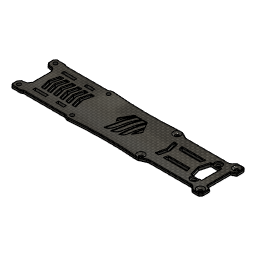
top_plate (Autodesk Fusion 360 design; units mm, degrees)
Autodesk Fusion 360 part; units mm, degrees
sketch "Sketch1" plane through (0, 0, 0) normal (0, 1, 0) x (1, 0, 0)
  line L0 (-47.713519, 13.1) -> (-47.713519, 11) construction
  line L1 (-41.213519, 13.1) -> (-41.213519, 11)
  line L2 (-56.590739, 11) -> (-67.090739, 11)
  line L3 (-67.090739, 11) -> (-67.090739, 13.1) construction
  line L4 (-47.713519, 11) -> (-47.713519, 13.1)
  line L5 (-41.213519, 11) -> (-47.713519, 11)
  line L6 (-56.590739, 11) -> (-67.090739, 11) construction
  line L7 (-67.090739, 13.1) -> (-56.590739, 13.1)
  line L8 (-47.713519, 13.1) -> (-41.213519, 13.1)
  line L9 (-56.590739, 13.1) -> (-56.590739, 11) construction
  line L10 (-41.213519, 11) -> (-41.213519, 13.1) construction
  line L11 (-41.213519, 13.1) -> (-47.713519, 13.1) construction
  line L12 (-47.713519, 11) -> (-41.213519, 11) construction
  line L13 (-56.590739, 13.1) -> (-56.590739, 11)
  line L14 (-67.090739, 11) -> (-67.090739, 13.1)
  line L15 (-67.090739, 13.1) -> (-56.590739, 13.1) construction
  line L16 (-70.174123, -18.17214) -> (-35.363156, -18.17214)
  arc A0 (25.451249, -18.878806) -> (-31.294288, -19.317303) centre (-0.303053, -357.951466) ccw
  line L17 (-78.946682, -19.052221) -> (-80.512717, -17.204486)
  line L18 (-80.512717, -17.204486) -> (-80.512717, -13.453934)
  line L19 (-80.512717, -13.453934) -> (-78.678868, -11.179487)
  line L20 (-72.154306, -19.052221) -> (-70.174123, -18.17214)
  line L21 (-78.678868, -11.179487) -> (-74.630702, -10.449798)
  line L22 (-41.21352, -11.000003) -> (-41.21352, -13.100003) construction
  line L23 (-47.71352, -11.000002) -> (-41.21352, -11.000003) construction
  line L24 (-41.21352, -13.100003) -> (-41.21352, -11.000003)
  line L25 (-47.71352, -13.100002) -> (-47.71352, -11.000002) construction
  line L26 (-56.59074, -11.000002) -> (-67.09074, -11.000001) construction
  line L27 (-41.21352, -13.100003) -> (-47.71352, -13.100002) construction
  line L28 (-56.59074, -13.100002) -> (-56.59074, -11.000002)
  line L29 (-67.09074, -13.100001) -> (-56.59074, -13.100002) construction
  line L30 (-67.09074, -13.100001) -> (-56.59074, -13.100002)
  line L31 (-47.71352, -11.000002) -> (-47.71352, -13.100002)
  line L32 (-41.21352, -11.000003) -> (-47.71352, -11.000002)
  line L33 (-56.59074, -11.000002) -> (-67.09074, -11.000001)
  line L34 (-56.59074, -13.100002) -> (-56.59074, -11.000002) construction
  line L35 (-47.71352, -13.100002) -> (-41.21352, -13.100003)
  line L36 (-67.09074, -11.000001) -> (-67.09074, -13.100001) construction
  line L37 (-67.09074, -11.000001) -> (-67.09074, -13.100001)
  circle A1 centre (-76.676945, -15.351861) radius 1.525
  line L38 (-74.630702, -10.449798) -> (-72.890045, -7.871569)
  line L39 (-78.946682, -19.052221) -> (-72.154306, -19.052221)
  line L40 (-72.890045, -7.871569) -> (-72.890045, 0.169525)
  circle A2 centre (-31.717186, 15.362679) radius 1.525
  circle A3 centre (-31.717186, -15.362679) radius 1.525
  circle A4 centre (26.228655, -15.29613) radius 1.525
  circle A5 centre (26.228655, 15.29613) radius 1.525
  arc A6 (-33.943222, -18.617483) -> (-35.363156, -18.17214) centre (-35.363156, -20.658473) ccw
  arc A7 (-33.943222, -18.617483) -> (-31.294288, -19.317303) centre (-31.658838, -15.33395) ccw
  line L41 (77.06033, 9.723206) -> (77.06033, 0)
  line L42 (80.674374, 17.200256) -> (80.667697, 11.53485)
  circle A8 centre (76.676945, 15.351861) radius 1.525
  line L43 (80.667697, 11.53485) -> (77.06033, 9.723206)
  line L44 (79.028958, 19.274953) -> (80.674374, 17.200256)
  line L45 (74.313283, 19.274953) -> (79.028958, 19.274953)
  line L46 (72.103018, 17.913723) -> (72.917518, 18.707378)
  line L47 (0, 0) -> (17, 0) construction
  arc A9 (-31.294288, 19.317303) -> (25.89772, 18.913013) centre (-0.303053, 357.951466) ccw
  arc A10 (-35.363156, 18.17214) -> (-33.943222, 18.617483) centre (-35.363156, 20.658473) ccw
  arc A11 (-31.294288, 19.317303) -> (-33.943222, 18.617483) centre (-31.658838, 15.33395) ccw
  line L48 (-70.174123, 18.17214) -> (-35.363156, 18.17214)
  line L49 (-72.154306, 19.052221) -> (-70.174123, 18.17214)
  line L50 (-72.890045, 7.871569) -> (-72.890045, -0.169525)
  line L51 (-78.678868, 11.179487) -> (-74.630702, 10.449798)
  line L52 (-80.512717, 13.453934) -> (-78.678868, 11.179487)
  line L53 (-74.630702, 10.449798) -> (-72.890045, 7.871569)
  circle A12 centre (-76.676945, 15.351861) radius 1.525
  line L54 (-78.946682, 19.052221) -> (-72.154306, 19.052221)
  line L55 (-80.512717, 17.204486) -> (-80.512717, 13.453934)
  line L56 (-78.946682, 19.052221) -> (-80.512717, 17.204486)
  line L57 (74.313283, -19.274953) -> (79.028958, -19.274953)
  line L58 (80.667697, -11.53485) -> (77.06033, -9.723206)
  line L59 (79.028958, -19.274953) -> (80.674374, -17.200256)
  line L60 (80.674374, -17.200256) -> (80.667697, -11.53485)
  line L61 (72.103018, -17.913723) -> (72.917518, -18.707378)
  circle A13 centre (76.676945, -15.351861) radius 1.525
  line L62 (77.06033, -9.723206) -> (77.06033, 0)
  line L63 (27.994774, 18.502613) -> (32.155418, 16.422291)
  line L64 (33.944272, 16) -> (68.977563, 16)
  line L65 (72.009935, 17.752225) -> (72.103018, 17.913723)
  line L66 (33.863514, -16) -> (68.977563, -16)
  line L67 (72.009935, -17.752225) -> (72.103018, -17.913723)
  line L68 (27.404322, -18.534068) -> (32.213389, -16.356227)
  arc A14 (27.994774, 18.502613) -> (25.89772, 18.913013) centre (26.20592, 14.924905) ccw
  arc A15 (32.155418, 16.422291) -> (33.944272, 16) centre (33.944272, 20) ccw
  arc A16 (33.863514, -16) -> (32.213389, -16.356227) centre (33.863514, -20) ccw
  arc A17 (25.451249, -18.878806) -> (27.404322, -18.534068) centre (25.754197, -14.890295) ccw
  arc A18 (68.977563, 16) -> (72.009935, 17.752225) centre (68.977563, 19.5) ccw
  arc A19 (72.009935, -17.752225) -> (68.977563, -16) centre (68.977563, -19.5) ccw
  arc A20 (74.313283, 19.274953) -> (72.917518, 18.707378) centre (74.313283, 17.274953) ccw
  arc A21 (72.917518, -18.707378) -> (74.313283, -19.274953) centre (74.313283, -17.274953) ccw
  point P0 (-76.676945, -15.351861)
  point P1 (-86.248614, -12.852519)
  point P2 (-76.676945, 15.351861)
  dimension "d36" = 10.5
  dimension "d37" = 2.1
  dimension "d38" = 6.5
  dimension "d39" = 2.1
  dimension "d132" = 4
  dimension "d144" = 4
  dimension "d145" = 4
  dimension "d146" = 4
  dimension "d147" = 4
  dimension "d148" = 3.5
  dimension "d149" = 3.5
  dimension "d150" = 2
  dimension "d151" = 2
  constraint horizontal L15
  constraint vertical L9
  constraint horizontal L6
  constraint vertical L3
  constraint horizontal L12
  constraint vertical L10
  constraint horizontal L11
  constraint vertical L0
  constraint horizontal L7
  constraint vertical L13
  constraint horizontal L2
  constraint vertical L14
  constraint horizontal L8
  constraint vertical L1
  constraint horizontal L5
  constraint vertical L4
  constraint vertical L40
  constraint horizontal L16
  constraint tangent L16 A6
  constraint tangent A0 A7
  constraint tangent A6 A7
  constraint coincident L47.start origin
  constraint horizontal L47
  constraint symmetric A0 L47 A9
  constraint symmetric A1 L47 A12
  constraint symmetric A6 L47 A10
  constraint symmetric A7 L47 A11
  constraint symmetric A8 L47 A13
  constraint vertical L62
  constraint tangent A9 A14
  constraint tangent L63 A14
  constraint tangent L63 A15
  constraint tangent L64 A15
  constraint tangent L68 A16
  constraint tangent L66 A16
  constraint tangent A0 A17
  constraint tangent L68 A17
  constraint tangent L65 A18
  constraint tangent L64 A18
  constraint tangent L67 A19
  constraint tangent L66 A19
  constraint tangent L46 A20
  constraint tangent L45 A20
  constraint tangent L61 A21
  constraint tangent L57 A21
  measures "d132" radius of A7
  measures "d144" radius of A14
  measures "d145" radius of A15
  measures "d146" radius of A16
  measures "d147" radius of A17
  measures "d148" radius of A18
  measures "d149" radius of A19
  measures "d150" radius of A20
  measures "d151" radius of A21
extrude "Extrude1" add sketch "Sketch1" along normal blind 2.5 contours L16 A0 L17 L18 L19 L20 L21 L38 L39 L40 A6 A7 L41 L42 L43 L44 L45 L46 A9 A10 A11 L48 L49 L50 L51 L52 L53 L54 L55 L56 L57 L58 L59 L60 L61 L62 L63 L64 L65 L66 L67 L68 A14 A15 A16 A17 A18 A19 A20 A21 picked at (45.595116, -5.333333)
sketch "Sketch2" plane through (0, 2.5, 0) normal (0, 1, 0) x (-1, 0, 0)
  line L0 (49.365614, -7.482923) -> (47.32507, -7.482923)
  line L1 (49.365614, 7.482923) -> (47.32507, 7.482923)
  line L2 (64.765331, -7.482923) -> (62.724788, -7.482923)
  line L3 (62.724788, 7.482923) -> (64.493676, 0)
  line L4 (57.769481, 7.482923) -> (59.538369, 0)
  line L5 (47.32507, 7.482923) -> (49.093958, 0)
  line L6 (47.32507, -7.482923) -> (49.093958, 0)
  line L7 (57.769481, -7.482923) -> (59.538369, 0)
  line L8 (57.769481, -7.482923) -> (59.538369, 0)
  line L9 (51.134502, 0) -> (49.365614, 7.482923)
  line L10 (47.32507, -7.482923) -> (49.093958, 0)
  line L11 (51.134502, 0) -> (49.365614, 7.482923)
  line L12 (62.724788, -7.482923) -> (64.493676, 0)
  line L13 (61.578913, 0) -> (59.810025, -7.482923)
  line L14 (49.365614, 7.482923) -> (47.32507, 7.482923)
  line L15 (66.534219, 0) -> (64.765331, -7.482923)
  line L16 (52.598933, -7.482923) -> (54.367821, 0)
  line L17 (51.134502, 0) -> (49.365614, -7.482923)
  line L18 (56.408365, 0) -> (54.639477, -7.482923)
  line L19 (51.134502, 0) -> (49.365614, -7.482923)
  line L20 (52.598933, -7.482923) -> (54.367821, 0)
  line L21 (47.32507, 7.482923) -> (49.093958, 0)
  line L22 (56.408365, 0) -> (54.639477, -7.482923)
  line L23 (61.578913, 0) -> (59.810025, -7.482923)
  line L24 (42.260502, 0) -> (17, 0) construction
  line L25 (59.810025, 7.482923) -> (57.769481, 7.482923)
  line L26 (59.810025, -7.482923) -> (57.769481, -7.482923)
  line L27 (64.765331, 7.482923) -> (62.724788, 7.482923)
  line L28 (61.578913, 0) -> (59.810025, 7.482923)
  line L29 (59.810025, 7.482923) -> (57.769481, 7.482923)
  line L30 (57.769481, 7.482923) -> (59.538369, 0)
  line L31 (59.810025, -7.482923) -> (57.769481, -7.482923)
  line L32 (49.365614, -7.482923) -> (47.32507, -7.482923)
  line L33 (56.408365, 0) -> (54.639477, 7.482923)
  line L34 (54.639477, 7.482923) -> (52.598933, 7.482923)
  line L35 (56.408365, 0) -> (54.639477, 7.482923)
  line L36 (66.534219, 0) -> (64.765331, 7.482923)
  line L37 (52.598933, 7.482923) -> (54.367821, 0)
  line L38 (54.639477, -7.482923) -> (52.598933, -7.482923)
  line L39 (61.578913, 0) -> (59.810025, 7.482923)
  line L40 (52.598933, 7.482923) -> (54.367821, 0)
  line L41 (54.639477, 7.482923) -> (52.598933, 7.482923)
  line L42 (54.639477, -7.482923) -> (52.598933, -7.482923)
  arc A0 (-25.451249, 18.878806) -> (31.294288, 19.317303) centre (0.303053, 357.951466) ccw
  line L43 (74.630702, 10.449798) -> (78.678868, 11.179487)
  line L44 (78.678868, 11.179487) -> (80.512717, 13.453934)
  line L45 (80.512717, 13.453934) -> (80.512717, 17.204486)
  line L46 (80.512717, 17.204486) -> (78.946682, 19.052221)
  line L47 (67.09074, 13.100001) -> (67.09074, 11.000001)
  line L48 (67.09074, 11.000001) -> (56.59074, 11.000002)
  line L49 (56.59074, 11.000002) -> (56.59074, 13.100002)
  line L50 (56.59074, 13.100002) -> (67.09074, 13.100001)
  line L51 (41.21352, 13.100003) -> (47.71352, 13.100002)
  line L52 (47.71352, 13.100002) -> (47.71352, 11.000002)
  line L53 (47.71352, 11.000002) -> (41.21352, 11.000003)
  line L54 (41.21352, 11.000003) -> (41.21352, 13.100003)
  line L55 (0, 0) -> (0, -25) construction
  line L56 (45.963858, 0) -> (44.19497, -7.482923)
  line L57 (42.154426, 7.482923) -> (43.923314, 0)
  line L58 (44.19497, -7.482923) -> (42.154426, -7.482923)
  line L59 (42.154426, 7.482923) -> (43.923314, 0)
  line L60 (38.921107, -7.482923) -> (36.880563, -7.482923)
  line L61 (44.19497, 7.482923) -> (42.154426, 7.482923)
  line L62 (36.880563, 7.482923) -> (38.649451, 0)
  line L63 (40.689995, 0) -> (38.921107, -7.482923)
  line L64 (40.689995, 0) -> (38.921107, 7.482923)
  line L65 (36.880563, -7.482923) -> (38.649451, 0)
  line L66 (45.963858, 0) -> (44.19497, 7.482923)
  line L67 (45.963858, 0) -> (44.19497, -7.482923)
  line L68 (38.921107, 7.482923) -> (36.880563, 7.482923)
  line L69 (42.154426, -7.482923) -> (43.923314, 0)
  line L70 (40.689995, 0) -> (38.921107, -7.482923)
  line L71 (40.689995, 0) -> (38.921107, 7.482923)
  line L72 (45.963858, 0) -> (44.19497, 7.482923)
  line L73 (38.921107, 7.482923) -> (36.880563, 7.482923)
  line L74 (36.880563, -7.482923) -> (38.649451, 0)
  line L75 (38.921107, -7.482923) -> (36.880563, -7.482923)
  line L76 (44.19497, -7.482923) -> (42.154426, -7.482923)
  line L77 (44.19497, 7.482923) -> (42.154426, 7.482923)
  line L78 (42.154426, -7.482923) -> (43.923314, 0)
  line L79 (36.880563, 7.482923) -> (38.649451, 0)
  line L80 (56.590739, -11) -> (67.090739, -11)
  line L81 (67.090739, -11) -> (67.090739, -13.1)
  line L82 (67.090739, -13.1) -> (56.590739, -13.1)
  line L83 (56.590739, -13.1) -> (56.590739, -11)
  line L84 (47.713519, -11) -> (47.713519, -13.1)
  line L85 (47.713519, -13.1) -> (41.213519, -13.1)
  line L86 (41.213519, -13.1) -> (41.213519, -11)
  line L87 (41.213519, -11) -> (47.713519, -11)
  line L88 (3.784933, -10.888484) -> (5.164029, -10.888484)
  line L89 (5.164029, -10.888484) -> (10.465412, -1.792331)
  line L90 (10.465412, -1.792331) -> (8.908366, 0.941707)
  spline S0 degree 2 poles (8.908366, 0.941707) (7.442966, -3.619944) (6.490839, -5.818435) knots 0 0 0 1 1 1
  spline S1 degree 2 poles (6.490839, -5.818435) (5.538712, -8.01694) (3.784933, -10.888484) knots 0 0 0 1 1 1
  line L91 (3.0098, -10.88842) -> (-0.824674, -10.88842)
  spline S2 degree 2 poles (-0.824674, -10.88842) (1.360907, -6.965735) (2.348646, -3.92432) knots 0 0 0 1 1 1
  spline S3 degree 3 poles (2.348646, -3.92432) (2.771725, -2.621651) (3.140209, -0.972131) (3.497406, 0.716522) knots 0 0 0 0 1 1 1 1
  spline S4 degree 2 poles (3.497406, 0.716522) (4.23037, 4.1815) (4.970387, 6.954955) knots 0 0 0 1 1 1
  spline S5 degree 2 poles (4.970387, 6.954955) (5.912838, 8.886413) (6.686031, 9.591534) knots 0 0 0 1 1 1
  spline S6 degree 2 poles (6.686031, 9.591534) (7.45921, 10.296651) (9.286239, 10.890851) knots 0 0 0 1 1 1
  spline S7 degree 2 poles (9.286239, 10.890851) (8.697628, 8.517032) (8.444231, 7.377107) knots 0 0 0 1 1 1
  spline S8 degree 3 poles (8.444231, 7.377107) (7.319167, 2.315979) (6.475945, -1.46655) (5.82273, -3.733217) knots 0 0 0 0 1 1 1 1
  spline S9 degree 2 poles (5.82273, -3.733217) (4.622239, -7.89888) (3.0098, -10.88842) knots 0 0 0 1 1 1
  line L92 (-5.475454, -10.888568) -> (-1.57567, -10.888568)
  spline S10 degree 2 poles (-1.57567, -10.888568) (-0.309354, -8.857824) (0.803309, -4.528704) knots 0 0 0 1 1 1
  spline S11 degree 3 poles (0.803309, -4.528704) (1.40458, -2.189429) (2.133696, 1.762827) (3.137408, 6.936551) knots 0 0 0 0 1 1 1 1
  spline S12 degree 2 poles (3.137408, 6.936551) (3.371965, 8.145592) (3.947428, 10.600128) knots 0 0 0 1 1 1
  spline S13 degree 2 poles (3.947428, 10.600128) (1.954848, 9.817553) (1.208318, 9.274906) knots 0 0 0 1 1 1
  spline S14 degree 2 poles (1.208318, 9.274906) (0.461787, 8.732257) (-0.413542, 6.936551) knots 0 0 0 1 1 1
  spline S15 degree 3 poles (-0.413542, 6.936551) (-1.94327, -0.721308) (-2.284933, -2.657156) (-2.760299, -4.305109) knots 0 0 0 0 1 1 1 1
  spline S16 degree 2 poles (-2.760299, -4.305109) (-3.726791, -7.655622) (-5.475454, -10.888568) knots 0 0 0 1 1 1
  line L93 (-5.931273, -10.089814) -> (-8.252962, -6.117535)
  spline S17 degree 2 poles (-8.252962, -6.117535) (-7.281055, -3.828239) (-6.709183, -1.384106) knots 0 0 0 1 1 1
  spline S18 degree 3 poles (-6.709183, -1.384106) (-6.653776, -1.1473) (-6.602886, -0.909225) (-6.555659, -0.670152) knots 0 0 0 0 1 1 1 1
  spline S19 degree 2 poles (-6.555659, -0.670152) (-5.82338, 3.035977) (-5.475431, 6.081951) knots 0 0 0 1 1 1
  spline S20 degree 2 poles (-5.475431, 6.081951) (-4.761037, 7.878925) (-4.217823, 8.34514) knots 0 0 0 1 1 1
  spline S21 degree 2 poles (-4.217823, 8.34514) (-3.67461, 8.811357) (-1.998782, 9.685931) knots 0 0 0 1 1 1
  spline S22 degree 2 poles (-1.998782, 9.685931) (-2.82745, 1.291461) (-3.650811, -2.849077) knots 0 0 0 1 1 1
  spline S23 degree 2 poles (-3.650811, -2.849077) (-4.474167, -6.989544) (-5.931273, -10.089814) knots 0 0 0 1 1 1
  line L94 (-10.780246, -1.792357) -> (-8.746198, -5.184925)
  spline S24 degree 2 poles (-8.746198, -5.184925) (-8.089469, -2.881961) (-7.835471, -1.200861) knots 0 0 0 1 1 1
  spline S25 degree 2 poles (-7.835471, -1.200861) (-7.581474, 0.480239) (-7.336445, 4.14564) knots 0 0 0 1 1 1
  spline S26 degree 2 poles (-7.336445, 4.14564) (-8.484273, 2.354181) (-9.058345, 1.364332) knots 0 0 0 1 1 1
  spline S27 degree 2 poles (-9.058345, 1.364332) (-9.632426, 0.374469) (-10.780246, -1.792357) knots 0 0 0 1 1 1
  line L95 (56.540739, -10.95) -> (67.140739, -10.95)
  line L96 (67.140739, -10.95) -> (67.140739, -13.15)
  line L97 (67.140739, -13.15) -> (56.540739, -13.15)
  line L98 (56.540739, -13.15) -> (56.540739, -10.95)
  line L99 (41.163519, -10.95) -> (47.763519, -10.95)
  line L100 (47.763519, -10.95) -> (47.763519, -13.15)
  line L101 (47.763519, -13.15) -> (41.163519, -13.15)
  line L102 (41.163519, -13.15) -> (41.163519, -10.95)
  line L103 (56.54074, 13.150002) -> (67.14074, 13.150001)
  line L104 (67.14074, 13.150001) -> (67.14074, 10.950001)
  line L105 (67.14074, 10.950001) -> (56.54074, 10.950002)
  line L106 (56.54074, 10.950002) -> (56.54074, 13.150002)
  line L107 (41.16352, 13.150003) -> (47.76352, 13.150002)
  line L108 (47.76352, 13.150002) -> (47.76352, 10.950002)
  line L109 (47.76352, 10.950002) -> (41.16352, 10.950003)
  line L110 (41.16352, 10.950003) -> (41.16352, 13.150003)
  line L111 (72.154306, -19.052221) -> (78.946682, -19.052221)
  line L112 (78.946682, -19.052221) -> (80.512717, -17.204486)
  line L113 (80.512717, -17.204486) -> (80.512717, -13.453934)
  line L114 (80.512717, -13.453934) -> (78.678868, -11.179487)
  line L115 (78.678868, -11.179487) -> (74.630702, -10.449798)
  line L116 (74.630702, -10.449798) -> (72.890045, -7.871569)
  line L117 (72.890045, -7.871569) -> (72.890045, 7.871569)
  line L118 (72.890045, 7.871569) -> (74.630702, 10.449798)
  line L119 (78.946682, 19.052221) -> (72.154306, 19.052221)
  line L120 (72.154306, 19.052221) -> (70.174123, 18.17214)
  line L121 (70.174123, 18.17214) -> (35.363156, 18.17214)
  arc A1 (33.943222, 18.617483) -> (35.363156, 18.17214) centre (35.363156, 20.658473) ccw
  arc A2 (33.943222, 18.617483) -> (31.294288, 19.317303) centre (31.658838, 15.33395) ccw
  line L122 (-77.06033, -9.723206) -> (-80.667697, -11.53485)
  line L123 (-80.667697, -11.53485) -> (-80.674374, -17.200256)
  line L124 (-80.674374, -17.200256) -> (-79.028958, -19.274953)
  line L125 (-79.028958, -19.274953) -> (-74.313283, -19.274953)
  line L126 (-72.917518, -18.707378) -> (-72.103018, -17.913723)
  arc A3 (31.294288, -19.317303) -> (-25.89772, -18.913013) centre (0.303053, -357.951466) ccw
  arc A4 (31.294288, -19.317303) -> (33.943222, -18.617483) centre (31.658838, -15.33395) ccw
  arc A5 (35.363156, -18.17214) -> (33.943222, -18.617483) centre (35.363156, -20.658473) ccw
  line L127 (35.363156, -18.17214) -> (70.174123, -18.17214)
  line L128 (70.174123, -18.17214) -> (72.154306, -19.052221)
  line L129 (-72.103018, 17.913723) -> (-72.917518, 18.707378)
  line L130 (-74.313283, 19.274953) -> (-79.028958, 19.274953)
  line L131 (-79.028958, 19.274953) -> (-80.674374, 17.200256)
  line L132 (-80.674374, 17.200256) -> (-80.667697, 11.53485)
  line L133 (-80.667697, 11.53485) -> (-77.06033, 9.723206)
  line L134 (-77.06033, 9.723206) -> (-77.06033, -9.723206)
  circle A6 centre (76.676945, 15.351861) radius 1.525
  circle A7 centre (-76.676945, -15.351861) radius 1.525
  circle A8 centre (-26.228655, -15.29613) radius 1.525
  circle A9 centre (31.717186, -15.362679) radius 1.525
  circle A10 centre (31.717186, 15.362679) radius 1.525
  circle A11 centre (-26.228655, 15.29613) radius 1.525
  circle A12 centre (76.676945, -15.351861) radius 1.525
  circle A13 centre (-76.676945, 15.351861) radius 1.525
  line L135 (-57.244978, 7.438362) -> (-38.408116, 7.438362)
  line L136 (-39.09255, 4.935443) -> (-56.560544, 4.935443)
  line L137 (-38.408116, -7.438362) -> (-57.244978, -7.438362)
  line L138 (-56.560544, -4.935443) -> (-39.09255, -4.935443)
  line L139 (-56.560544, 4.935443) -> (-57.244978, 7.438362)
  line L140 (-57.244978, -7.438362) -> (-56.560544, -4.935443)
  line L141 (-38.408116, 7.438362) -> (-39.09255, 4.935443)
  line L142 (-39.09255, -4.935443) -> (-38.408116, -7.438362)
  line L143 (-35.348965, 0) -> (-33.580077, 7.482923)
  line L144 (-31.539534, 7.482923) -> (-33.308422, 0)
  line L145 (-33.580077, 7.482923) -> (-31.539534, 7.482923)
  line L146 (-33.580077, -7.482923) -> (-35.348965, 0)
  line L147 (-33.308422, 0) -> (-31.539534, -7.482923)
  line L148 (-31.539534, -7.482923) -> (-33.580077, -7.482923)
  line L149 (-27.404322, 18.534068) -> (-32.213389, 16.356227)
  line L150 (-33.863514, 16) -> (-68.977563, 16)
  line L151 (-72.009935, 17.752225) -> (-72.103018, 17.913723)
  line L152 (-72.103018, -17.913723) -> (-72.009935, -17.752225)
  line L153 (-68.977563, -16) -> (-33.944272, -16)
  line L154 (-32.155418, -16.422291) -> (-27.994774, -18.502613)
  arc A14 (-25.451249, 18.878806) -> (-27.404322, 18.534068) centre (-25.754197, 14.890295) ccw
  arc A15 (-33.863514, 16) -> (-32.213389, 16.356227) centre (-33.863514, 20) ccw
  arc A16 (-32.155418, -16.422291) -> (-33.944272, -16) centre (-33.944272, -20) ccw
  arc A17 (-27.994774, -18.502613) -> (-25.89772, -18.913013) centre (-26.20592, -14.924905) ccw
  arc A18 (-72.917518, 18.707378) -> (-74.313283, 19.274953) centre (-74.313283, 17.274953) ccw
  arc A19 (-74.313283, -19.274953) -> (-72.917518, -18.707378) centre (-74.313283, -17.274953) ccw
  arc A20 (-68.977563, -16) -> (-72.009935, -17.752225) centre (-68.977563, -19.5) ccw
  arc A21 (-72.009935, 17.752225) -> (-68.977563, 16) centre (-68.977563, 19.5) ccw
  point P0 (66.429305, 0)
  point P1 (66.429305, 0)
  dimension "d110" = -0.05
  dimension "d111" = -0.05
  dimension "d112" = -0.05
  dimension "d113" = -0.05
  constraint horizontal L2
  constraint parallel L12 L15
  constraint horizontal L26
  constraint parallel L7 L13
  constraint horizontal L31
  constraint parallel L8 L23
  constraint horizontal L38
  constraint parallel L16 L22
  constraint horizontal L42
  constraint parallel L18 L20
  constraint horizontal L32
  constraint parallel L6 L19
  constraint horizontal L0
  constraint parallel L10 L17
  constraint coincident L55.start origin
  constraint horizontal L76
  constraint parallel L56 L69
  constraint horizontal L58
  constraint parallel L67 L78
  constraint horizontal L75
  constraint parallel L63 L74
  constraint horizontal L60
  constraint parallel L65 L70
sketch "Sketch3" plane through (0, 2.5, 0) normal (0, 1, 0) x (-1, 0, 0)
  arc A0 (-25.451249, 18.878806) -> (31.294288, 19.317303) centre (0.303053, 357.951466) ccw
  line L0 (74.630702, 10.449798) -> (78.678868, 11.179487)
  line L1 (78.678868, 11.179487) -> (80.512717, 13.453934)
  line L2 (80.512717, 13.453934) -> (80.512717, 17.204486)
  line L3 (80.512717, 17.204486) -> (78.946682, 19.052221)
  line L4 (67.09074, 13.100001) -> (67.09074, 11.000001)
  line L5 (67.09074, 11.000001) -> (56.59074, 11.000002)
  line L6 (56.59074, 11.000002) -> (56.59074, 13.100002)
  line L7 (56.59074, 13.100002) -> (67.09074, 13.100001)
  line L8 (41.21352, 13.100003) -> (47.71352, 13.100002)
  line L9 (47.71352, 13.100002) -> (47.71352, 11.000002)
  line L10 (47.71352, 11.000002) -> (41.21352, 11.000003)
  line L11 (41.21352, 11.000003) -> (41.21352, 13.100003)
  line L12 (56.590739, -11) -> (67.090739, -11)
  line L13 (67.090739, -11) -> (67.090739, -13.1)
  line L14 (67.090739, -13.1) -> (56.590739, -13.1)
  line L15 (56.590739, -13.1) -> (56.590739, -11)
  line L16 (47.713519, -11) -> (47.713519, -13.1)
  line L17 (47.713519, -13.1) -> (41.213519, -13.1)
  line L18 (41.213519, -13.1) -> (41.213519, -11)
  line L19 (41.213519, -11) -> (47.713519, -11)
  line L20 (72.154306, -19.052221) -> (78.946682, -19.052221)
  line L21 (78.946682, -19.052221) -> (80.512717, -17.204486)
  line L22 (80.512717, -17.204486) -> (80.512717, -13.453934)
  line L23 (80.512717, -13.453934) -> (78.678868, -11.179487)
  line L24 (78.678868, -11.179487) -> (74.630702, -10.449798)
  line L25 (74.630702, -10.449798) -> (72.890045, -7.871569)
  line L26 (72.890045, -7.871569) -> (72.890045, 7.871569)
  line L27 (72.890045, 7.871569) -> (74.630702, 10.449798)
  line L28 (78.946682, 19.052221) -> (72.154306, 19.052221)
  line L29 (72.154306, 19.052221) -> (70.174123, 18.17214)
  line L30 (70.174123, 18.17214) -> (35.363156, 18.17214)
  arc A1 (33.943222, 18.617483) -> (35.363156, 18.17214) centre (35.363156, 20.658473) ccw
  arc A2 (33.943222, 18.617483) -> (31.294288, 19.317303) centre (31.658838, 15.33395) ccw
  line L31 (-77.06033, -9.723206) -> (-80.667697, -11.53485)
  line L32 (-80.667697, -11.53485) -> (-80.674374, -17.200256)
  line L33 (-80.674374, -17.200256) -> (-79.028958, -19.274953)
  line L34 (-79.028958, -19.274953) -> (-74.313283, -19.274953)
  line L35 (-72.917518, -18.707378) -> (-72.103018, -17.913723)
  arc A3 (31.294288, -19.317303) -> (-25.89772, -18.913013) centre (0.303053, -357.951466) ccw
  arc A4 (31.294288, -19.317303) -> (33.943222, -18.617483) centre (31.658838, -15.33395) ccw
  arc A5 (35.363156, -18.17214) -> (33.943222, -18.617483) centre (35.363156, -20.658473) ccw
  line L36 (35.363156, -18.17214) -> (70.174123, -18.17214)
  line L37 (70.174123, -18.17214) -> (72.154306, -19.052221)
  line L38 (-72.103018, 17.913723) -> (-72.917518, 18.707378)
  line L39 (-74.313283, 19.274953) -> (-79.028958, 19.274953)
  line L40 (-79.028958, 19.274953) -> (-80.674374, 17.200256)
  line L41 (-80.674374, 17.200256) -> (-80.667697, 11.53485)
  line L42 (-80.667697, 11.53485) -> (-77.06033, 9.723206)
  line L43 (-77.06033, 9.723206) -> (-77.06033, -9.723206)
  circle A6 centre (76.676945, 15.351861) radius 1.525
  circle A7 centre (-76.676945, -15.351861) radius 1.525
  circle A8 centre (-26.228655, -15.29613) radius 1.525
  circle A9 centre (31.717186, -15.362679) radius 1.525
  circle A10 centre (31.717186, 15.362679) radius 1.525
  circle A11 centre (-26.228655, 15.29613) radius 1.525
  circle A12 centre (76.676945, -15.351861) radius 1.525
  circle A13 centre (-76.676945, 15.351861) radius 1.525
  line L44 (-27.404322, 18.534068) -> (-32.213389, 16.356227)
  line L45 (-33.863514, 16) -> (-68.977563, 16)
  line L46 (-72.009935, 17.752225) -> (-72.103018, 17.913723)
  line L47 (-72.103018, -17.913723) -> (-72.009935, -17.752225)
  line L48 (-68.977563, -16) -> (-33.944272, -16)
  line L49 (-32.155418, -16.422291) -> (-27.994774, -18.502613)
  arc A14 (-25.451249, 18.878806) -> (-27.404322, 18.534068) centre (-25.754197, 14.890295) ccw
  arc A15 (-33.863514, 16) -> (-32.213389, 16.356227) centre (-33.863514, 20) ccw
  arc A16 (-32.155418, -16.422291) -> (-33.944272, -16) centre (-33.944272, -20) ccw
  arc A17 (-27.994774, -18.502613) -> (-25.89772, -18.913013) centre (-26.20592, -14.924905) ccw
  arc A18 (-72.917518, 18.707378) -> (-74.313283, 19.274953) centre (-74.313283, 17.274953) ccw
  arc A19 (-74.313283, -19.274953) -> (-72.917518, -18.707378) centre (-74.313283, -17.274953) ccw
  arc A20 (-68.977563, -16) -> (-72.009935, -17.752225) centre (-68.977563, -19.5) ccw
  arc A21 (-72.009935, 17.752225) -> (-68.977563, 16) centre (-68.977563, 19.5) ccw
sketch "Sketch4" plane through (0, 2.5, 0) normal (0, 1, 0) x (-1, 0, 0)
  line L0 (67.09074, 13.100001) -> (67.09074, 11.000001)
  line L1 (67.09074, 11.000001) -> (56.59074, 11.000002)
  line L2 (56.59074, 11.000002) -> (56.59074, 13.100002)
  line L3 (56.59074, 13.100002) -> (67.09074, 13.100001)
  line L4 (41.21352, 13.100003) -> (47.71352, 13.100002)
  line L5 (47.71352, 13.100002) -> (47.71352, 11.000002)
  line L6 (47.71352, 11.000002) -> (41.21352, 11.000003)
  line L7 (41.21352, 11.000003) -> (41.21352, 13.100003)
  line L8 (74.630702, 10.449798) -> (78.678868, 11.179487)
  line L9 (78.678868, 11.179487) -> (80.512717, 13.453934)
  line L10 (80.512717, 13.453934) -> (80.512717, 17.204486)
  line L11 (80.512717, 17.204486) -> (78.946682, 19.052221)
  arc A0 (-25.451249, 18.878806) -> (31.294288, 19.317303) centre (0.303053, 357.951466) ccw
  line L12 (56.590739, -11) -> (67.090739, -11)
  line L13 (67.090739, -11) -> (67.090739, -13.1)
  line L14 (67.090739, -13.1) -> (56.590739, -13.1)
  line L15 (56.590739, -13.1) -> (56.590739, -11)
  line L16 (47.713519, -11) -> (47.713519, -13.1)
  line L17 (47.713519, -13.1) -> (41.213519, -13.1)
  line L18 (41.213519, -13.1) -> (41.213519, -11)
  line L19 (41.213519, -11) -> (47.713519, -11)
  line L20 (72.154306, -19.052221) -> (78.946682, -19.052221)
  line L21 (78.946682, -19.052221) -> (80.512717, -17.204486)
  line L22 (80.512717, -17.204486) -> (80.512717, -13.453934)
  line L23 (80.512717, -13.453934) -> (78.678868, -11.179487)
  line L24 (78.678868, -11.179487) -> (74.630702, -10.449798)
  line L25 (74.630702, -10.449798) -> (72.890045, -7.871569)
  line L26 (72.890045, -7.871569) -> (72.890045, 7.871569)
  line L27 (72.890045, 7.871569) -> (74.630702, 10.449798)
  line L28 (78.946682, 19.052221) -> (72.154306, 19.052221)
  line L29 (72.154306, 19.052221) -> (70.174123, 18.17214)
  line L30 (70.174123, 18.17214) -> (35.363156, 18.17214)
  arc A1 (33.943222, 18.617483) -> (35.363156, 18.17214) centre (35.363156, 20.658473) ccw
  arc A2 (33.943222, 18.617483) -> (31.294288, 19.317303) centre (31.658838, 15.33395) ccw
  line L31 (-77.06033, -9.723206) -> (-80.667697, -11.53485)
  line L32 (-80.667697, -11.53485) -> (-80.674374, -17.200256)
  line L33 (-80.674374, -17.200256) -> (-79.028958, -19.274953)
  line L34 (-79.028958, -19.274953) -> (-74.313283, -19.274953)
  line L35 (-72.917518, -18.707378) -> (-72.103018, -17.913723)
  arc A3 (31.294288, -19.317303) -> (-25.89772, -18.913013) centre (0.303053, -357.951466) ccw
  arc A4 (31.294288, -19.317303) -> (33.943222, -18.617483) centre (31.658838, -15.33395) ccw
  arc A5 (35.363156, -18.17214) -> (33.943222, -18.617483) centre (35.363156, -20.658473) ccw
  line L36 (35.363156, -18.17214) -> (70.174123, -18.17214)
  line L37 (70.174123, -18.17214) -> (72.154306, -19.052221)
  line L38 (-72.103018, 17.913723) -> (-72.917518, 18.707378)
  line L39 (-74.313283, 19.274953) -> (-79.028958, 19.274953)
  line L40 (-79.028958, 19.274953) -> (-80.674374, 17.200256)
  line L41 (-80.674374, 17.200256) -> (-80.667697, 11.53485)
  line L42 (-80.667697, 11.53485) -> (-77.06033, 9.723206)
  line L43 (-77.06033, 9.723206) -> (-77.06033, -9.723206)
  circle A6 centre (76.676945, 15.351861) radius 1.525
  circle A7 centre (-76.676945, -15.351861) radius 1.525
  circle A8 centre (-26.228655, -15.29613) radius 1.525
  circle A9 centre (31.717186, -15.362679) radius 1.525
  circle A10 centre (31.717186, 15.362679) radius 1.525
  circle A11 centre (-26.228655, 15.29613) radius 1.525
  circle A12 centre (76.676945, -15.351861) radius 1.525
  circle A13 centre (-76.676945, 15.351861) radius 1.525
  line L44 (-70.347842, 8.00136) -> (-62.171638, 8.00136)
  line L45 (-62.171638, 8.00136) -> (-62.171638, -7.99864)
  line L46 (-62.171638, -7.99864) -> (-70.347842, -7.99864)
  line L47 (-70.347842, -7.99864) -> (-70.347842, 8.00136)
  line L48 (-70.347842, 8.00136) -> (-62.171638, -7.99864) construction
  line L49 (-62.171638, 8.00136) -> (-70.347842, -7.99864) construction
  line L50 (-66.25974, 0.00136) -> (-66.25974, 10.25136) construction
  circle A14 centre (-66.25974, 10.25136) radius 1.5
  line L51 (-66.25974, 0.00136) -> (-68.381403, 0.00136) construction
  arc A15 (-68.150847, 7.872763) -> (-67.537373, 9.089722) centre (-68.175066, 8.648079) ccw
  arc A16 (-65.14647, 9.109265) -> (-64.491693, 7.787577) centre (-64.452409, 8.630074) ccw
  line L52 (-27.404322, 18.534068) -> (-32.213389, 16.356227)
  line L53 (-33.863514, 16) -> (-68.977563, 16)
  line L54 (-72.009935, 17.752225) -> (-72.103018, 17.913723)
  line L55 (-72.103018, -17.913723) -> (-72.009935, -17.752225)
  line L56 (-68.977563, -16) -> (-33.944272, -16)
  line L57 (-32.155418, -16.422291) -> (-27.994774, -18.502613)
  arc A17 (-25.451249, 18.878806) -> (-27.404322, 18.534068) centre (-25.754197, 14.890295) ccw
  arc A18 (-33.863514, 16) -> (-32.213389, 16.356227) centre (-33.863514, 20) ccw
  arc A19 (-32.155418, -16.422291) -> (-33.944272, -16) centre (-33.944272, -20) ccw
  arc A20 (-27.994774, -18.502613) -> (-25.89772, -18.913013) centre (-26.20592, -14.924905) ccw
  arc A21 (-72.917518, 18.707378) -> (-74.313283, 19.274953) centre (-74.313283, 17.274953) ccw
  arc A22 (-74.313283, -19.274953) -> (-72.917518, -18.707378) centre (-74.313283, -17.274953) ccw
  arc A23 (-68.977563, -16) -> (-72.009935, -17.752225) centre (-68.977563, -19.5) ccw
  arc A24 (-72.009935, 17.752225) -> (-68.977563, 16) centre (-68.977563, 19.5) ccw
  line L58 (-62.171638, 8.00136) -> (-59.908914, 0.070882)
  line L59 (-59.908914, 0.070882) -> (-62.171638, -7.99864)
  circle A25 centre (-66.25974, 10.25136) radius 3.1
  circle A26 centre (-66.25974, -10.24864) radius 3.1
  arc A27 (-64.491693, -7.784856) -> (-65.14647, -9.106544) centre (-64.452409, -8.627354) ccw
  arc A28 (-67.537373, -9.087001) -> (-68.150847, -7.870042) centre (-68.175066, -8.645358) ccw
  circle A29 centre (-66.25974, -10.24864) radius 1.5
  point P0 (-66.25974, 0.00136)
  point P1 (-66.25974, -10.24864)
  dimension "d136" = 16
  dimension "d139" = 3
  dimension "d155" = 6.2
  dimension "d159" = 10.25
  dimension "d160" = 16
  constraint horizontal L44
  constraint perpendicular L44 L45
  constraint parallel L45 L47
  constraint perpendicular L44 L50
  constraint perpendicular L50 L51
  constraint concentric A14 A25
  constraint symmetric A14 L51 A29
  constraint symmetric L51 A15 A28
  constraint symmetric L51 A16 A27
  constraint symmetric L51 A25 A26
  measures "d139" diameter of A14
  measures "d155" diameter of A25
hole "Hole2" at (26.228655, 2.5, -15.29613) at (26.228655, 2.5, 15.29613) at (76.676945, 2.5, 15.351861) at (76.676945, 2.5, -15.351861) direction (0, -1, 0) diameter 3.2 depth 4.760684 tip angle 118 countersink diameter 6.2 countersink angle 90
extrude "Extrude4" cut sketch "Sketch2" against normal blind 4.341 contours L95 L96 L97 L98 | L99 L100 L101 L102 | L103 L104 L105 L106 | L107 L108 L109 L110 | L135 L136 L139 L141 | L137 L138 L140 L142 | L143 L144 L145 L146 L147 L148 picked at (60.090739, -13.133333) picked at (43.380186, -13.133333) picked at (63.59074, 10.966668) picked at (45.546853, 10.966669) picked at (-44.915215, 6.604056) picked at (-44.915215, -6.604056) picked at (-32.809344, -4.988615)
extrude "Extrude6" cut sketch "Sketch2" against normal blind 10.279 contours L0 L1 L5 L6 L9 L10 L11 L14 L17 L19 L21 L32 | L2 L3 L12 L15 L27 L36 | L4 L7 L8 L13 L23 L25 L26 L28 L29 L30 L31 L39 | L16 L18 L20 L22 L33 L34 L35 L37 L38 L40 L41 L42 | L56 L57 L58 L59 L61 L66 L67 L69 L72 L76 L77 L78 | L60 L62 L63 L64 L65 L68 L70 L71 L73 L74 L75 L79 picked at (48.594881, -4.988615) picked at (63.994598, -4.988615) picked at (59.039292, -4.988615) picked at (53.868744, -4.988615) picked at (44.694047, -2.494308) picked at (38.150374, -4.988615)
extrude "Extrude8" cut sketch "Sketch4" against normal blind 3.556 contours L44 L45 L46 L47 A25 A26 | L44 A25 | L46 A26 | L45 L58 L59 | A14 | A29 picked at (-63.18505, 2.445517) picked at (-66.411569, 7.720483) picked at (-66.411569, -7.717762) picked at (-61.417397, 0.024534) picked at (-66.794006, 10.642276) picked at (-66.794006, -9.857724)
chamfer "Chamfer17" distance 0.5 angle 45 96 edges at (-2.930683, 2.5, 17.912279) (26.44949, 2.5, 18.829402) (29.808855, 2.5, 17.445147) (33.019445, 2.5, 16.090071) (51.420538, 2.5, 16) (70.728675, 2.5, 16.469554) (72.056476, 2.5, 17.832974) (-52.76864, 2.5, 18.17214) (-34.619089, 2.5, 18.286087) (-32.680541, 2.5, 19.201265) (-2.930683, 0, 17.912279) (-32.680541, 0, 19.201265) (-34.619089, 0, 18.286087) (-52.76864, 0, 18.17214) (72.056476, 0, 17.832974) (70.728675, 0, 16.469554) (51.420538, 0, 16) (33.019445, 0, 16.090071) (29.808855, 0, 17.445147) (26.44949, 0, 18.829402) (-2.706799, 2.5, -17.910623) (-32.680541, 2.5, -19.201265) (-34.619089, 2.5, -18.286087) (-52.76864, 2.5, -18.17214) (72.056476, 2.5, -17.832974) (70.728675, 2.5, -16.469554) (51.460918, 2.5, -16) (33.025261, 2.5, -16.107004) (30.075096, 2.5, -17.462452) (26.974159, 2.5, -18.850437) (-2.706799, 0, -17.910623) (26.974159, 0, -18.850437) (30.075096, 0, -17.462452) (33.025261, 0, -16.107004) (51.460918, 0, -16) (70.728675, 0, -16.469554) (72.056476, 0, -17.832974) (-52.76864, 0, -18.17214) (-34.619089, 0, -18.286087) (-32.680541, 0, -19.201265) (-71.164214, 2.5, 18.61218) (-75.550494, 2.5, 19.052221) (-79.729699, 2.5, 18.128354) (-80.512717, 2.5, 15.32921) (-79.595793, 2.5, 12.31671) (-76.654785, 2.5, 10.814642) (-73.760374, 2.5, 9.160683) (-72.890045, 2.5, 0) (-73.760374, 2.5, -9.160683) (-76.654785, 2.5, -10.814642) (-79.595793, 2.5, -12.31671) (-80.512717, 2.5, -15.32921) (-79.729699, 2.5, -18.128354) (-75.550494, 2.5, -19.052221) (-71.164214, 2.5, -18.61218) (-75.550494, 0, -19.052221) (-71.164214, 0, -18.61218) (-79.729699, 0, -18.128354) (-80.512717, 0, -15.32921) (-79.595793, 0, -12.31671) (-76.654785, 0, -10.814642) (-73.760374, 0, -9.160683) (-72.890045, 0, 0) (-73.760374, 0, 9.160683) (-76.654785, 0, 10.814642) (-79.595793, 0, 12.31671) (-80.512717, 0, 15.32921) (-79.729699, 0, 18.128354) (-75.550494, 0, 19.052221) (-71.164214, 0, 18.61218) (72.510268, 0, 18.31055) (73.559907, 0, 19.127634) (76.671121, 0, 19.274953) (79.851666, 0, 18.237605) (73.559907, 2.5, 19.127634) (76.671121, 2.5, 19.274953) (72.510268, 2.5, 18.31055) (79.851666, 2.5, 18.237605) (80.671035, 0, 14.367553) (80.671035, 2.5, 14.367553) (78.864013, 0, 10.629028) (78.864013, 2.5, 10.629028) (77.06033, 2.5, 0) (77.06033, 0, 0) (78.864013, 0, -10.629028) (78.864013, 2.5, -10.629028) (80.671035, 2.5, -14.367553) (80.671035, 0, -14.367553) (79.851666, 0, -18.237605) (79.851666, 2.5, -18.237605) (76.671121, 0, -19.274953) (72.510268, 0, -18.31055) (73.559907, 0, -19.127634) (76.671121, 2.5, -19.274953) (73.559907, 2.5, -19.127634) (72.510268, 2.5, -18.31055)
chamfer "Chamfer18" distance 0.5 angle 45 55 edges at (66.25974, 2.5, -7.99864) (70.347842, 2.5, 0.00136) (66.25974, 2.5, 8.00136) (61.040276, 2.5, 4.036121) (61.040276, 2.5, -3.963879) (47.826547, 2.5, -7.438362) (56.902761, 2.5, -6.186903) (47.826547, 2.5, -4.935443) (38.750333, 2.5, -6.186903) (47.826547, 2.5, 4.935443) (56.902761, 2.5, 6.186903) (47.826547, 2.5, 7.438362) (38.750333, 2.5, 6.186903) (34.464521, 2.5, 3.741461) (34.464521, 2.5, -3.741461) (32.559806, 2.5, -7.482923) (32.423978, 2.5, -3.741461) (32.423978, 2.5, 3.741461) (32.559806, 2.5, 7.482923) (-37.765007, 2.5, -3.741461) (-37.900835, 2.5, -7.482923) (-39.805551, 2.5, -3.741461) (-39.805551, 2.5, 3.741461) (-37.765007, 2.5, 3.741461) (-37.900835, 2.5, 7.482923) (-43.03887, 2.5, 3.741461) (-43.03887, 2.5, -3.741461) (-43.174698, 2.5, -7.482923) (-45.079414, 2.5, -3.741461) (-45.079414, 2.5, 3.741461) (-43.174698, 2.5, 7.482923) (-48.209514, 2.5, 3.741461) (-48.209514, 2.5, -3.741461) (-48.345342, 2.5, -7.482923) (-50.250058, 2.5, -3.741461) (-50.250058, 2.5, 3.741461) (-48.345342, 2.5, 7.482923) (-53.619205, 2.5, -7.482923) (-53.483377, 2.5, -3.741461) (-53.483377, 2.5, 3.741461) (-53.619205, 2.5, 7.482923) (-55.523921, 2.5, 3.741461) (-55.523921, 2.5, -3.741461) (-58.653925, 2.5, -3.741461) (-58.789753, 2.5, -7.482923) (-60.694469, 2.5, -3.741461) (-58.653925, 2.5, 3.741461) (-58.789753, 2.5, 7.482923) (-60.694469, 2.5, 3.741461) (-63.609232, 2.5, 3.741461) (-63.609232, 2.5, -3.741461) (-63.745059, 2.5, -7.482923) (-65.649775, 2.5, -3.741461) (-65.649775, 2.5, 3.741461) (-63.745059, 2.5, 7.482923)
extrude "Extrude9" cut sketch "Sketch4" against normal blind 1 contours L44 L45 L46 L47 A25 A26 | L44 A25 | L46 A26 picked at (-63.18505, 2.445517) picked at (-66.377729, 8.252759) picked at (-66.377729, -8.250038)
extrude "Extrude10" cut sketch "Sketch2" against normal blind 0.5 contours L88 L89 L90 S0 S1 | L91 S2 S3 S4 S5 S6 S7 S8 S9 | L92 S10 S11 S12 S13 S14 S15 S16 | L93 S17 S18 S19 S20 S21 S22 S23 | L94 S24 S25 S26 S27 picked at (8.621539, -2.22302) picked at (5.921456, 1.453471) picked at (-0.790177, -0.632421) picked at (-3.708341, 4.306268) picked at (-9.120638, -2.726048)
